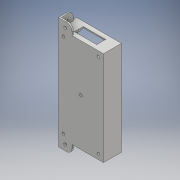
# Autodesk Inventor part: OLED_holder
Saved by Autodesk Inventor 2018 (Build 220112000, 112)
## iProperties
Created: 2018-04-29
Part Number: OLED_holder
Material: 一般
Document SubType Name: Modeling
Designer: izumi
Density: 1 g/cm^3
Appearance: 既定
Author: izumi
Autodesk Inventor part; units mm, degrees
ref_plane "YZ Plane" through (0, 0, 0) normal (1, 0, 0) x (0, 1, 0)
ref_plane "XZ Plane" through (0, 0, 0) normal (0, 1, 0) x (-1, 0, 0)
ref_plane "XY Plane" through (0, 0, 0) normal (0, 0, 1) x (1, 0, 0)
sketch "本体面" plane through (0, 0, 0) normal (0, 1, 0) x (-1, 0, 0)
  line L0 (20, 42) -> (-20, 42)
  line L1 (-20, 42) -> (-20, -42)
  line L2 (-20, -42) -> (20, -42)
  line L3 (20, -42) -> (20, 42)
  line L4 (20, 0) -> (-20, 0) construction
  line L5 (0, 42) -> (0, -42) construction
  point P0 (0, 0)
  point P1 (0, 0)
  dimension "d0" = 84
  dimension "d1" = 40
  constraints: 12 end point, 5 midpoint, 2 parallel, 2 perpendicular, 1 coincident, 1 horizontal
  measures "d0" distance of L2.end L0.start
  measures "d1" distance of L0.start L0.end
extrude "本体" add sketch "本体面" against normal blind 16
sketch "背羽形状" plane through (0, -16, 0) normal (0, -1, 0) x (1, 0, 0)
  line L0 (-20, -50) -> (-13, -50)
  line L1 (-8, -45) -> (-8, 45)
  line L2 (-13, 50) -> (-20, 50)
  line L3 (-20, 50) -> (-20, -50)
  line L4 (-20, 42) -> (-20, -42) projected
  arc A0 (-13, -50) -> (-8, -45) centre (-13, -45) ccw
  arc A1 (-8, 45) -> (-13, 50) centre (-13, 45) ccw
  point P0 (0, 0)
  point P1 (-8, 50)
  point P2 (-8, -50)
  point P3 (-20, 0)
  point P4 (-20, 50)
  point P5 (-20, -50)
  dimension "d94" = 100
  dimension "d95" = 12
  dimension "d128" = 5
  constraints: 8 end point, 4 point on circle, 4 point on line, 4 tangent, 2 centre point, 2 midpoint, 2 parallel, 1 equal radius, 1 horizontal, 1 perpendicular
  measures "d94" distance of L2.end L0.start
  measures "d95" distance of L0.start point (-8, -50)
  measures "d128" radius of A0
extrude "背羽" add sketch "背羽形状" against normal blind 1.2
sketch "上羽形状" plane through (-20, 0, -42) normal (-1, 0, 0) x (0, 0, 1)
  line L0 (92, -16) -> (-8, -16)
  line L1 (-8, -16) -> (-8, -9)
  line L2 (-3, -4) -> (87, -4)
  line L3 (92, -9) -> (92, -16)
  line L4 (92, -16) -> (-8, -16) projected
  arc A0 (92, -9) -> (87, -4) centre (87, -9) ccw
  arc A1 (-3, -4) -> (-8, -9) centre (-3, -9) ccw
  point P0 (42, 0)
  point P1 (-8, -4)
  point P2 (92, -4)
  point P3 (42, -16)
  dimension "d122" = 100
  dimension "d123" = 12
  dimension "d124" = 5
  dimension "d125" = 5
  constraints: 8 end point, 4 point on circle, 4 point on line, 4 tangent, 2 centre point, 2 midpoint, 2 parallel, 1 horizontal, 1 perpendicular
  measures "d122" distance of point (-8, -4) point (92, -4)
  measures "d123" distance of L0.end point (-8, -4)
  measures "d124" radius of A0
  measures "d125" radius of A1
extrude "上羽" add sketch "上羽形状" against normal blind 1.2
sketch "空洞上面" plane through (0, 0, 0) normal (0, 1, 0) x (1, 0, 0)
  line L0 (-19, -41) -> (19, -41)
  line L1 (19, -41) -> (19, 41)
  line L2 (19, 41) -> (-19, 41)
  line L3 (-19, 41) -> (-19, -41)
  line L4 (-19, 0) -> (19, 0) construction
  line L5 (0, -41) -> (0, 41) construction
  point P0 (0, 0)
  point P1 (0, 0)
  dimension "d4" = 82
  dimension "d5" = 38
  constraints: 12 end point, 5 midpoint, 2 parallel, 1 coincident, 1 horizontal, 1 perpendicular
  measures "d4" distance of L2.end L0.start
  measures "d5" distance of L0.start L0.end
extrude "空洞上" cut sketch "空洞上面" against normal blind 6
sketch "空洞下面" plane through (0, -6, 0) normal (0, 1, 0) x (1, 0, 0)
  line L0 (-13, -40) -> (13, -40)
  line L1 (18, -35) -> (18, 35)
  line L2 (13, 40) -> (-13, 40)
  line L3 (-18, 35) -> (-18, -35)
  line L4 (-18, 0) -> (18, 0) construction
  line L5 (0, -40) -> (0, 40) construction
  line L6 (-14, -35) -> (-18, -35)
  line L7 (-13, -36) -> (-13, -40)
  line L8 (14, -35) -> (18, -35)
  line L9 (13, -36) -> (13, -40)
  line L10 (-14, 35) -> (-18, 35)
  line L11 (-13, 36) -> (-13, 40)
  line L12 (14, 35) -> (18, 35)
  line L13 (13, 36) -> (13, 40)
  arc A0 (-13, -36) -> (-14, -35) centre (-14, -36) ccw
  arc A1 (14, -35) -> (13, -36) centre (14, -36) ccw
  arc A2 (-14, 35) -> (-13, 36) centre (-14, 36) ccw
  arc A3 (13, 36) -> (14, 35) centre (14, 36) ccw
  point P0 (0, 0)
  point P1 (0, 0)
  point P2 (-13, -35)
  point P3 (13, -35)
  point P4 (-13, 35)
  point P5 (13, 35)
  dimension "d10" = 36
  dimension "d11" = 80
  dimension "d12" = 5
  dimension "d13" = 5
  dimension "d14" = 5
  dimension "d15" = 5
  dimension "d16" = 5
  dimension "d17" = 5
  dimension "d18" = 5
  dimension "d19" = 5
  dimension "d20" = 1
  constraints: 28 end point, 9 perpendicular, 8 point on circle, 8 point on line, 8 tangent, 6 midpoint, 4 centre point, 3 equal radius, 3 horizontal, 2 parallel, 1 coincident
  measures "d10" distance of L4.start L4.end
  measures "d11" distance of L5.start L5.end
  measures "d12" distance of L3.end point (-13, -35)
  measures "d13" distance of L0.start point (-13, -35)
  measures "d14" distance of L0.end point (13, -35)
  measures "d15" distance of L1.start point (13, -35)
  measures "d16" distance of L3.start point (-13, 35)
  measures "d17" distance of L2.end point (-13, 35)
  measures "d18" distance of L2.start point (13, 35)
  measures "d19" distance of L1.end point (13, 35)
  measures "d20" radius of A0
extrude "空洞下" cut sketch "空洞下面" against normal blind 8
sketch "取付穴位置" plane through (0, -6, 0) normal (0, 1, 0) x (1, 0, 0)
  line L0 (0, 37.5) -> (0, -37.5) construction
  line L1 (-15.5, -37.5) -> (15.5, -37.5) construction
  line L2 (-15.5, 37.5) -> (15.5, 37.5) construction
  point P0 (0, 0)
  point P1 (0, 0)
  dimension "d26" = 75
  dimension "d27" = 31
  dimension "d28" = 31
  constraints: 6 end point, 5 coincident, 3 midpoint, 2 horizontal, 1 vertical
  measures "d26" distance of L0.end L0.start
  measures "d27" distance of L1.start L1.end
  measures "d28" distance of L2.start L2.end
hole "取付穴" at (-15.5, -6, 37.5) at (15.5, -6, 37.5) at (-15.5, -6, -37.5) at (15.5, -6, -37.5) direction (0, -1, 0) diameter 2.4 depth 20 tip angle 118
sketch "ケーブル穴右形状" plane through (20, 0, -42) normal (0, 0, -1) x (-1, 0, 0)
  line L0 (0, 0) -> (20, 0) construction
  line L1 (20, 0) -> (20, -8) construction
  line L2 (20, -4) -> (20, -12) construction
  line L3 (10, -4) -> (30, -4)
  line L4 (30, -4) -> (30, -12)
  line L5 (30, -12) -> (10, -12)
  line L6 (10, -12) -> (10, -4)
  line L7 (10, -4) -> (30, -12) construction
  line L8 (30, -4) -> (10, -12) construction
  point P0 (20, 0)
  point P1 (24, -8)
  dimension "d76" = 20
  dimension "d155" = 8
  dimension "d156" = 20
  constraints: 18 end point, 4 midpoint, 2 horizontal, 2 parallel, 2 perpendicular, 1 coincident
  measures "d76" distance of L0.start L0.end
  measures "d155" distance of L3.end L4.end
  measures "d156" distance of L4.end L5.end
extrude "ケーブル穴右" cut sketch "ケーブル穴右形状" against normal blind 5
sketch "ケーブル穴左形状" plane through (-20, 0, 42) normal (0, 0, 1) x (1, 0, 0)
  line L0 (0, 0) -> (20, 0) construction
  line L1 (20, 0) -> (20, -8) construction
  line L2 (20, -4) -> (20, -12) construction
  line L3 (10, -4) -> (30, -4) projected
  line L4 (10, -12) -> (30, -12)
  line L5 (30, -12) -> (30, -4)
  line L6 (30, -4) -> (10, -4)
  line L7 (10, -4) -> (10, -12)
  line L8 (10, -12) -> (30, -4) construction
  line L9 (30, -12) -> (10, -4) construction
  point P0 (20, 0)
  dimension "d98" = 20
  dimension "d99" = 8
  dimension "d101" = 8
  dimension "d157" = 20
  constraints: 18 end point, 3 midpoint, 2 coincident, 2 horizontal, 2 parallel, 2 perpendicular
  measures "d98" distance of L0.start L0.end
  measures "d99" distance of L0.end L1.end
  measures "d101" distance of L2.start L2.end
  measures "d157" distance of L4.start L4.end
extrude "ケーブル穴左" cut sketch "ケーブル穴左形状" against normal blind 5
sketch "上穴位置" plane through (-20, 0, -42) normal (-1, 0, 0) x (0, 0, 1)
  line L0 (42, -16) -> (42, -10) construction
  line L1 (92, -16) -> (-8, -16) construction
  line L2 (86.45, -10) -> (-2.45, -10) construction
  point P0 (42, 0)
  dimension "d129" = 6
  dimension "d130" = 88.9
  constraints: 4 end point, 3 coincident, 2 midpoint, 1 horizontal, 1 vertical
  measures "d129" distance of L0.end L0.start
  measures "d130" distance of L2.start L2.end
hole "上穴" at (-20, -10, 44.45) at (-20, -10, 0) at (-20, -10, -44.45) direction (1, 0, 0) diameter 2.5 depth 8 tip angle 118
sketch "背穴位置" plane through (0, -16, 0) normal (0, -1, 0) x (1, 0, 0)
  line L0 (-20, 0) -> (20, 0) construction
  line L1 (-20, 50) -> (-20, -50) construction
  line L2 (-14, -45) -> (-14, 45) construction
  line L3 (20, -42) -> (20, 42) construction
  point P0 (0, 0)
  point P1 (-14, 0)
  point P2 (0, 0)
  dimension "d139" = 90
  dimension "d147" = 6
  constraints: 4 end point, 3 coincident, 3 midpoint, 1 horizontal, 1 point on line, 1 vertical
  measures "d139" distance of L2.start L2.end
  measures "d147" distance between parallel lines of L1 L2
hole "背穴" at (-14, -16, -45) at (-14, -16, 45) at (0, -16, 0) direction (0, 1, 0) diameter 2.5 depth 8 tip angle 118
